output_shaft_cover v13 (Autodesk Fusion 360 design; units mm, degrees)
Autodesk Fusion 360 part; units mm, degrees
note: some values were not read from the file. Set by a fixed rule: which face or edge a step refers to.
sketch "Sketch1" plane through (0, 0, 0) normal (0, 0, 1) x (1, 0, 0)
  circle A0 centre (0, 0) radius 27
  line L0 (0, 0) -> (0, 27) construction
  circle A1 centre (0, 27) radius 2.25
  circle A2 centre (0, 27) radius 3.5
  circle A3 centre (0, 0) radius 31.5
  circle A4 centre (0, 0) radius 18.5
  circle A5 centre (0, 0) radius 17.5
  circle A6 centre (-13.5, 23.3827) radius 2.25
  circle A7 centre (-13.5, 23.3827) radius 3.5
  circle A8 centre (-23.3827, 13.5) radius 2.25
  circle A9 centre (-23.3827, 13.5) radius 3.5
  circle A10 centre (-27, 0) radius 2.25
  circle A11 centre (-27, 0) radius 3.5
  circle A12 centre (-23.3827, -13.5) radius 2.25
  circle A13 centre (-23.3827, -13.5) radius 3.5
  circle A14 centre (-13.5, -23.3827) radius 2.25
  circle A15 centre (-13.5, -23.3827) radius 3.5
  circle A16 centre (0, -27) radius 2.25
  circle A17 centre (0, -27) radius 3.5
  circle A18 centre (13.5, -23.3827) radius 2.25
  circle A19 centre (13.5, -23.3827) radius 3.5
  circle A20 centre (23.3827, -13.5) radius 2.25
  circle A21 centre (23.3827, -13.5) radius 3.5
  circle A22 centre (27, 0) radius 2.25
  circle A23 centre (27, 0) radius 3.5
  circle A24 centre (23.3827, 13.5) radius 2.25
  circle A25 centre (23.3827, 13.5) radius 3.5
  circle A26 centre (13.5, 23.3827) radius 2.25
  circle A27 centre (13.5, 23.3827) radius 3.5
  circle A28 centre (0, 0) radius 21.5
  dimension "d1" = 54
  dimension "d2" = 4.5
  dimension "d3" = 7
  dimension "d4" = 37
  dimension "d5" = 35
  dimension "d6" = 63
  dimension "d8" = 360
  dimension "d25" = 43
  constraint coincident A0.centre L0.start
  constraint coincident A0 L0.end
  constraint vertical L0
  constraint coincident L0.end A1.centre
  constraint concentric A1 A2
  constraint concentric A4 A5
  constraint concentric A0 A28
  measures "d1" diameter of A0
  measures "d2" diameter of A1
  measures "d3" diameter of A2
  measures "d4" diameter of A4
  measures "d5" diameter of A5
  measures "d6" diameter of A3
  measures "d25" diameter of A28
extrude "Extrude1" add sketch "Sketch1" along normal blind 9 contours A0 A2 A7 A9 A11 A13 A15 A17 A19 A21 A23 A25 A27 | A3 | A4 | A28
extrude "Extrude2" cut sketch "Sketch1" along normal blind 7 contours A4
extrude "Extrude3" add sketch "Sketch1" along normal blind 2 contours A0 A22 A23 | A0 A22 A23 | A0 A24 A25 | A0 A24 A25 | A0 A20 A21 | A0 A20 A21 | A0 A26 A27 | A0 A26 A27 | A0 A18 A19 | A0 A18 A19 | A0 A1 A2 | A0 A1 A2 | A0 A16 A17 | A0 A16 A17 | A0 A6 A7 | A0 A6 A7 | A0 A14 A15 | A0 A14 A15 | A0 A8 A9 | A0 A8 A9 | A0 A12 A13 | A0 A12 A13 | A0 A10 A11 | A0 A10 A11
extrude "Extrude4" add sketch "Sketch1" against normal blind 6 contours A0 A22 A23 | A0 A22 A23 | A0 A2 A7 A9 A11 A13 A15 A17 A19 A21 A23 A25 A27 | A0 A24 A25 | A0 A24 A25 | A0 A20 A21 | A0 A20 A21 | A0 A26 A27 | A0 A26 A27 | A0 A18 A19 | A0 A18 A19 | A0 A1 A2 | A0 A1 A2 | A0 A16 A17 | A0 A16 A17 | A0 A6 A7 | A0 A6 A7 | A0 A14 A15 | A0 A14 A15 | A0 A8 A9 | A0 A8 A9 | A0 A12 A13 | A0 A12 A13 | A0 A10 A11 | A0 A10 A11 | A3
extrude "Extrude5" cut 48 faces at (-20.3124, -13.3261, 2) (16.5703, 23.5566, 2) (26.453, 13.6739, 2) (26.453, -13.3261, 2) (30.0703, 0.1739, 2) (3.0619, -26.7143, 2) (-10.4381, 23.6684, 2) (-10.4297, -23.2088, 2) (16.5619, -23.097, 2) (2.8826, 25.9289, 2) (-20.3124, 13.6739, 2) (-23.9297, 0.1739, 2) (-20.3124, -13.3261, 2) (16.5703, 23.5566, 2) (26.453, 13.6739, 2) (26.453, -13.3261, 2) (30.0703, 0.1739, 2) (3.0619, -26.7143, 2) (-10.4381, 23.6684, 2) (-10.4297, -23.2088, 2) (16.5619, -23.097, 2) (2.8826, 25.9289, 2) (-20.3124, 13.6739, 2) (-23.9297, 0.1739, 2) (2.8826, 25.9289, 2) (-10.4381, 23.6684, 2) (-20.3124, 13.6739, 2) (-23.9297, 0.1739, 2) (-20.3124, -13.3261, 2) (-10.4297, -23.2088, 2) (3.0619, -26.7143, 2) (16.5619, -23.097, 2) (26.453, -13.3261, 2) (26.453, 13.6739, 2) (30.0703, 0.1739, 2) (16.5703, 23.5566, 2) (-20.3124, -13.3261, 2) (16.5703, 23.5566, 2) (26.453, 13.6739, 2) (26.453, -13.3261, 2) (30.0703, 0.1739, 2) (3.0619, -26.7143, 2) (-10.4381, 23.6684, 2) (-10.4297, -23.2088, 2) (16.5619, -23.097, 2) (2.8826, 25.9289, 2) (-20.3124, 13.6739, 2) (-23.9297, 0.1739, 2) along direction (0, 0, -1) blind 6
sketch "Sketch2" plane through (0, 0, -6) normal (0, 0, -1) x (1, 0, 0)
  circle A0 centre (0, -27) radius 2.25
  circle A1 centre (13.5, -23.3827) radius 2.25
  circle A2 centre (13.5, 23.3827) radius 2.25
  circle A3 centre (-27, 0) radius 2.25
  circle A4 centre (-23.3827, -13.5) radius 2.25
  circle A5 centre (0, 27) radius 2.25
  circle A6 centre (23.3827, -13.5) radius 2.25
  circle A7 centre (23.3827, 13.5) radius 2.25
  circle A8 centre (-23.3827, 13.5) radius 2.25
  circle A9 centre (-13.5, -23.3827) radius 2.25
  circle A10 centre (-13.5, 23.3827) radius 2.25
  circle A11 centre (27, 0) radius 2.25
  circle A12 centre (0, 0) radius 31.5
  line L0 (0, 0) -> (-40, 0) construction
  circle A13 centre (-35, 0) radius 2.75
  line L1 (0, 0) -> (0, -30) construction
  line L2 (-31.1006, -5) -> (-40, -5)
  line L3 (-40, -5) -> (-40, 5)
  line L4 (-40, 5) -> (-31.1006, 5)
  line L5 (31.1006, -5) -> (40, -5)
  line L6 (40, -5) -> (40, 5)
  circle A14 centre (35, 0) radius 2.75
  line L7 (40, 5) -> (31.1006, 5)
  circle A15 centre (0, 0) radius 21.5
  dimension "d19" = 5.5
  dimension "d20" = 35
  dimension "d21" = 10
  dimension "d22" = 5
  constraint coincident A12.centre L0.start
  constraint horizontal L0
  constraint coincident L0 A13.centre
  constraint perpendicular L0 L1
  constraint coincident A12 L2.start
  constraint parallel L0 L2
  constraint perpendicular L0 L3
  constraint coincident A12 L4.end
  constraint perpendicular L3 L4
  constraint symmetric L0 L2 L4
  constraint symmetric A13 L1 A14
  constraint symmetric L1 L2.start L5.start
  constraint symmetric L1 L2.end L5.end
  constraint symmetric L1 L3.end L6.end
  constraint symmetric L1 L4.end L7.end
  measures "d19" diameter of A13
  measures "d20" distance of A12.centre A13.centre
  measures "d21" distance of L2.end L3.end
  measures "d22" distance of A13.centre L3
extrude "Extrude6" [suppressed]
